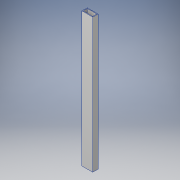
# Autodesk Inventor part: 29in 2x1
Saved by Autodesk Inventor 2018 (Build 220112000, 112)
## iProperties
Created: 2018-01-13
Part Number: 29in 2x1
Material: Aluminum 6061
Document SubType Name: Modeling
Designer: maste
Density: 2.7 g/cm^3
Appearance: Aluminum - Flat
Author: maste
Autodesk Inventor part; units mm, degrees
ref_plane "YZ Plane" through (0, 0, 0) normal (1, 0, 0) x (0, 1, 0)
ref_plane "XZ Plane" through (0, 0, 0) normal (0, 1, 0) x (-1, 0, 0)
ref_plane "XY Plane" through (0, 0, 0) normal (0, 0, 1) x (1, 0, 0)
sketch "Sketch1" plane through (0, 0, 0) normal (0, 1, 0) x (-1, 0, 0)
  line L0 (0, 0) -> (-50.8, 0)
  line L1 (-50.8, 0) -> (-50.8, -25.4)
  line L2 (-50.8, -25.4) -> (0, -25.4)
  line L3 (0, -25.4) -> (0, 0)
  line L4 (-3.175, -22.225) -> (-47.625, -22.225)
  line L5 (-47.625, -22.225) -> (-47.625, -3.175)
  line L6 (-47.625, -3.175) -> (-3.175, -3.175)
  line L7 (-3.175, -3.175) -> (-3.175, -22.225)
  dimension "d0" = 25.4
  dimension "d1" = 50.8
  dimension "d2" = 3.175
  dimension "d3" = 3.175
  dimension "d4" = 3.175
  dimension "d5" = 3.175
  constraints: 16 end point, 4 parallel, 2 horizontal, 2 perpendicular
  measures "d0" distance of L0.end L1.end
  measures "d1" distance of L1.end L2.end
  measures "d2" distance between parallel lines of L2 L4
  measures "d3" distance between parallel lines of L0 L6
  measures "d4" distance between parallel lines of L1 L5
  measures "d5" distance between parallel lines of L3 L7
extrude "Extrusion1" add sketch "Sketch1" along normal blind 736.6
sketch "Sketch2" plane through (0, 736.6, 0) normal (0, 1, 0) x (1, 0, 0)
  line L0 (-32.6558, 46.2997) -> (107.3615, 46.2997)
  line L1 (107.3615, 46.2997) -> (107.3615, -26.8404)
  line L2 (107.3615, -26.8404) -> (-32.6558, -26.8404)
  line L3 (-32.6558, -26.8404) -> (-32.6558, 46.2997)
  point P0 (0, 0)
  constraints: 8 end point, 2 parallel, 1 horizontal, 1 perpendicular
extrude "Extrusion2" cut sketch "Sketch2" against normal blind 101.6
body "Solid1"
